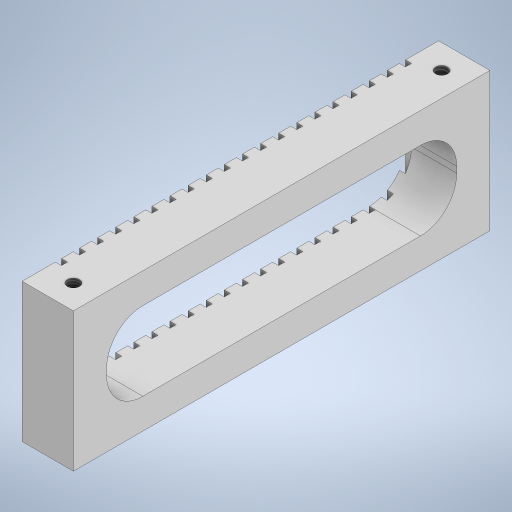
# Autodesk Inventor part: RectangularHolderWall
Saved by Autodesk Inventor 2024 (Build 280153000, 153)
## iProperties
Created: 2023-08-14
Part Number: RectangularHolderWall
Material: Generic
Document SubType Name: Modeling
Designer: ewinden
Density: 1 g/cm^3
Appearance: Default
Author: ewinden
Autodesk Inventor part; units mm, degrees
ref_plane "YZ Plane" through (0, 0, 0) normal (1, 0, 0) x (0, 1, 0)
ref_plane "XZ Plane" through (0, 0, 0) normal (0, 1, 0) x (-1, 0, 0)
ref_plane "XY Plane" through (0, 0, 0) normal (0, 0, 1) x (1, 0, 0)
sketch "Sketch1" plane through (0, 0, 0) normal (0, 1, 0) x (-1, 0, 0)
  line L0 (0, 0) -> (8.5, 0)
  line L1 (8.5, -69) -> (0, -69)
  line L2 (0, -69) -> (0, 0)
  line L3 (8.5, 0) -> (8.5, -5.5)
  line L4 (8.5, -69) -> (8.5, -65.5)
  line L5 (8.5, -5.5) -> (7.5, -5.5)
  line L6 (7.5, -5.5) -> (7.5, -6.5)
  line L7 (7.5, -6.5) -> (8.5, -6.5)
  line L8 (8.5, -6.5) -> (8.5, -8.5)
  line L9 (8.5, -8.5) -> (7.5, -8.5)
  line L10 (7.5, -8.5) -> (7.5, -9.5)
  line L11 (7.5, -9.5) -> (8.5, -9.5)
  line L12 (8.5, -9.5) -> (8.5, -11.5)
  line L13 (8.5, -11.5) -> (7.5, -11.5)
  line L14 (7.5, -11.5) -> (7.5, -12.5)
  line L15 (7.5, -12.5) -> (8.5, -12.5)
  line L16 (8.5, -12.5) -> (8.5, -14.5)
  line L17 (8.5, -14.5) -> (7.5, -14.5)
  line L18 (7.5, -14.5) -> (7.5, -15.5)
  line L19 (7.5, -15.5) -> (8.5, -15.5)
  line L20 (8.5, -15.5) -> (8.5, -17.5)
  line L21 (8.5, -17.5) -> (7.5, -17.5)
  line L22 (7.5, -17.5) -> (7.5, -18.5)
  line L23 (7.5, -18.5) -> (8.5, -18.5)
  line L24 (8.5, -18.5) -> (8.5, -20.5)
  line L25 (8.5, -20.5) -> (7.5, -20.5)
  line L26 (7.5, -20.5) -> (7.5, -21.5)
  line L27 (7.5, -21.5) -> (8.5, -21.5)
  line L28 (8.5, -21.5) -> (8.5, -23.5)
  line L29 (8.5, -23.5) -> (7.5, -23.5)
  line L30 (7.5, -23.5) -> (7.5, -24.5)
  line L31 (7.5, -24.5) -> (8.5, -24.5)
  line L32 (8.5, -24.5) -> (8.5, -26.5)
  line L33 (8.5, -26.5) -> (7.5, -26.5)
  line L34 (7.5, -26.5) -> (7.5, -27.5)
  line L35 (7.5, -27.5) -> (8.5, -27.5)
  line L36 (8.5, -27.5) -> (8.5, -29.5)
  line L37 (8.5, -29.5) -> (7.5, -29.5)
  line L38 (7.5, -29.5) -> (7.5, -30.5)
  line L39 (7.5, -30.5) -> (8.5, -30.5)
  line L40 (8.5, -30.5) -> (8.5, -32.5)
  line L41 (8.5, -32.5) -> (7.5, -32.5)
  line L42 (7.5, -32.5) -> (7.5, -33.5)
  line L43 (7.5, -33.5) -> (8.5, -33.5)
  line L44 (8.5, -33.5) -> (8.5, -35.5)
  line L45 (8.5, -35.5) -> (7.5, -35.5)
  line L46 (7.5, -35.5) -> (7.5, -36.5)
  line L47 (7.5, -36.5) -> (8.5, -36.5)
  line L48 (8.5, -36.5) -> (8.5, -38.5)
  line L49 (8.5, -38.5) -> (7.5, -38.5)
  line L50 (7.5, -38.5) -> (7.5, -39.5)
  line L51 (7.5, -39.5) -> (8.5, -39.5)
  line L52 (8.5, -39.5) -> (8.5, -41.5)
  line L53 (8.5, -41.5) -> (7.5, -41.5)
  line L54 (7.5, -41.5) -> (7.5, -42.5)
  line L55 (7.5, -42.5) -> (8.5, -42.5)
  line L56 (8.5, -42.5) -> (8.5, -44.5)
  line L57 (8.5, -44.5) -> (7.5, -44.5)
  line L58 (7.5, -44.5) -> (7.5, -45.5)
  line L59 (7.5, -45.5) -> (8.5, -45.5)
  line L60 (8.5, -45.5) -> (8.5, -47.5)
  line L61 (8.5, -47.5) -> (7.5, -47.5)
  line L62 (7.5, -47.5) -> (7.5, -48.5)
  line L63 (7.5, -48.5) -> (8.5, -48.5)
  line L64 (8.5, -48.5) -> (8.5, -50.5)
  line L65 (8.5, -50.5) -> (7.5, -50.5)
  line L66 (7.5, -50.5) -> (7.5, -51.5)
  line L67 (7.5, -51.5) -> (8.5, -51.5)
  line L68 (8.5, -51.5) -> (8.5, -53.5)
  line L69 (8.5, -53.5) -> (7.5, -53.5)
  line L70 (7.5, -53.5) -> (7.5, -54.5)
  line L71 (7.5, -54.5) -> (8.5, -54.5)
  line L72 (8.5, -54.5) -> (8.5, -56.5)
  line L73 (8.5, -56.5) -> (7.5, -56.5)
  line L74 (7.5, -56.5) -> (7.5, -57.5)
  line L75 (7.5, -57.5) -> (8.5, -57.5)
  line L76 (8.5, -57.5) -> (8.5, -59.5)
  line L77 (8.5, -59.5) -> (7.5, -59.5)
  line L78 (7.5, -59.5) -> (7.5, -60.5)
  line L79 (7.5, -60.5) -> (8.5, -60.5)
  line L80 (8.5, -60.5) -> (8.5, -62.5)
  line L81 (8.5, -62.5) -> (7.5, -62.5)
  line L82 (7.5, -62.5) -> (7.5, -63.5)
  line L83 (7.5, -63.5) -> (8.5, -63.5)
  line L84 (8.5, -63.5) -> (8.5, -65.5)
  dimension "d0" = 8.5
  dimension "d1" = 69
  dimension "d2" = 1
  dimension "d3" = 2
  dimension "d6" = 3
  dimension "d11" = 5.5
  constraints: 170 end point, 2 horizontal, 2 perpendicular, 1 coincident, 1 parallel, 1 vertical, 171 other
  measures "d0" distance of L0.start L0.end
  measures "d1" distance of L0.end L1.start
  measures "d2" distance of L3.end L5.end
  measures "d3" distance of L7.end L8.end
  measures "d6" distance of L3.end L9.start
  measures "d11" distance of L0.end L3.end
extrude "Extrusion1" add sketch "Sketch1" along normal blind 23
sketch "Sketch2" plane through (0, 0, 0) normal (1, 0, 0) x (0, 0, -1)
  line L0 (5.5, 0) -> (5.5, 23) projected
  line L1 (63.5, 0) -> (63.5, 23) projected
  line L2 (11.5, 5) -> (57.5, 5)
  line L3 (63.5, 11) -> (63.5, 12)
  line L4 (57.5, 18) -> (11.5, 18)
  line L5 (5.5, 12) -> (5.5, 11)
  line L6 (0, 23) -> (69, 23) projected
  line L7 (0, 0) -> (69, 0) projected
  arc A0 (11.5, 18) -> (5.5, 12) centre (11.5, 12) ccw
  arc A1 (5.5, 11) -> (11.5, 5) centre (11.5, 11) ccw
  arc A2 (57.5, 5) -> (63.5, 11) centre (57.5, 11) ccw
  arc A3 (63.5, 12) -> (57.5, 18) centre (57.5, 12) ccw
  point P0 (5.5, 5)
  point P1 (63.5, 18)
  dimension "d14" = 5
  dimension "d15" = 5
  dimension "d16" = 6
  constraints: 8 end point, 8 point on circle, 8 tangent, 6 point on line, 4 centre point, 3 equal radius, 2 parallel, 1 horizontal, 1 perpendicular
  measures "d14" distance between parallel lines of L6 L4
  measures "d15" distance between parallel lines of L7 L2
  measures "d16" radius of A0
extrude "Extrusion2" cut sketch "Sketch2" against normal blind 10 contours L0 A0 L4 A3 L1 A2 L2 A1
sketch "Sketch3" plane through (0, 23, 0) normal (0, 1, 0) x (1, 0, 0)
  circle A0 centre (-4, 4) radius 1
  circle A1 centre (-4, 65) radius 1
  line L0 (-8.5, 0) -> (0, 0) construction
  line L1 (-4, 0) -> (-4, 4) construction
  line L2 (-4, 4) -> (0, 4) construction
  line L3 (0, 0) -> (0, 69) construction
  line L4 (-4, 65) -> (0, 65) construction
  line L5 (-4, 65) -> (-4, 69) construction
  line L6 (0, 69) -> (-8.5, 69) construction
  dimension "d19" = 2
  dimension "d20" = 4
  constraints: 8 end point, 4 point on line, 3 equal length, 2 centre point, 2 vertical, 1 equal radius, 1 parallel, 1 perpendicular
  measures "d19" diameter of A0
  measures "d20" distance of L1.start L1.end
extrude "Extrusion3" cut sketch "Sketch3" against normal blind 8
thread "Thread1" size "M2x0.4" class "6H" standard "ANSI Metric M Profile" full length
thread "Thread2" size "4-40 UNC" class "2B" standard "ANSI Unified Screw Threads" full length
body "Solid1"
